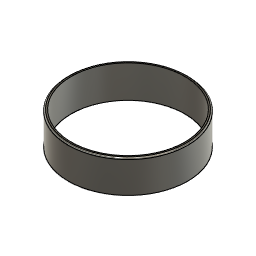
side v9 (Autodesk Fusion 360 design; units mm, degrees)
Autodesk Fusion 360 part; units mm, degrees
sketch "Sketch3" plane through (0, 0, 0) normal (0, 1, 0) x (1, 0, 0)
  circle A0 centre (0, 0) radius 40.3
  circle A1 centre (0, 0) radius 42.3
  line L0 (30, -20) -> (-30, -20)
  line L1 (-30, -20) -> (-30, 20)
  line L2 (-30, 20) -> (30, 20)
  line L3 (30, 20) -> (30, -20)
  line L4 (30, -20) -> (-30, 20) construction
  line L5 (-30, -20) -> (30, 20) construction
  dimension "d13" = 80.6
  dimension "d14" = 2
  dimension "d34" = 60
  dimension "d35" = 40
  constraint coincident A0.centre A1.centre
  constraint perpendicular L0 L1
  constraint parallel L0 L2
  constraint parallel L1 L3
  constraint horizontal L0
  constraint coincident L4 A0.centre
  constraint coincident L5 A0.centre
  measures "d13" diameter of A0
  measures "d34" distance of L1.end L2.end
  measures "d35" distance of L0.end L1.end
extrude "Extrude3" add sketch "Sketch3" along normal blind 21 contours A1
sketch "Sketch4" plane through (0, 0, 0) normal (0, 0, 1) x (1, 0, 0)
  line L0 (-49.5, 21) -> (-47.3, 21)
  line L1 (49.5, 21) -> (47.3, 21)
  line L2 (-47.3, 21) -> (-47.3, 25.1334)
  line L3 (47.3, 21) -> (47.3, 25.1334)
  line L4 (47.3, 27) -> (47.3, 25)
  arc A0 (47.3, 25) -> (-47.3, 25) centre (0, -131.3064) ccw
  line L5 (47.3, 21) -> (45.3, 21)
  line L6 (45.3, 21) -> (45.3, 25.5913)
  line L7 (-47.3, 21) -> (-45.3, 21)
  line L8 (-45.3, 21) -> (-45.3, 25.5913)
  arc A1 (0, 32) -> (-47.3, 25) centre (0, -131.3064) ccw
  line L9 (0, 32) -> (0, 34)
  arc A2 (45.4965, 27.5344) -> (-45.4965, 27.5344) centre (0, -129.3064) ccw
  arc A3 (-45.4965, 27.5344) -> (-47.3, 25.1334) centre (-44.8, 25.1334) ccw
  arc A4 (47.3, 25.1334) -> (45.4965, 27.5344) centre (44.8, 25.1334) ccw
  line L10 (0, 21) -> (-2.5, 21)
  line L11 (-2.5, 21) -> (-2.5, 31.9809)
  line L12 (0, 21) -> (0, 32)
  line L13 (-42, 21) -> (-39.8, 21)
  line L14 (42, 21) -> (39.8, 21)
  line L15 (39.8, 21) -> (39.8, 27.0759)
  line L16 (-39.8, 21) -> (-39.8, 27.0759)
  line L17 (-39.8, 21) -> (-37.8, 21)
  line L18 (-37.8, 21) -> (-37.8, 27.5651)
  line L19 (37.8, 21) -> (37.8, 27.5651)
  line L20 (37.8, 21) -> (39.8, 21)
  line L21 (-39.8, 27.0759) -> (-39.8, 29.0759)
  line L22 (39.8, 27.0759) -> (39.8, 29.0759)
  line L23 (-39.8, 27.0759) -> (0, 27.0759)
  line L24 (0, 27.0759) -> (0, 34)
  point P0 (-47.3, 27)
  dimension "d17" = 2.2
  dimension "d18" = 2.2
  dimension "d19" = 6
  dimension "d20" = 6
  dimension "d22" = 2
  dimension "d23" = 2
  dimension "d24" = 2
  dimension "d25" = 2
  dimension "d26" = 2
  dimension "d27" = 2.5
  dimension "d28" = 2.5
  dimension "d36" = 2.2
  dimension "d37" = 2.2
  dimension "d38" = 2
  dimension "d39" = 2
  constraint horizontal L0
  constraint horizontal L1
  constraint perpendicular L0 L2
  constraint perpendicular L1 L3
  constraint coincident L2 A0.end
  constraint coincident A1.start A0
  constraint perpendicular L3 L5
  constraint coincident A0 L6.end
  constraint perpendicular L5 L6
  constraint perpendicular L2 L7
  constraint coincident A0 L8.end
  constraint perpendicular L7 L8
  constraint vertical L9
  constraint coincident L9.end A2
  constraint coincident P0 L2
  constraint coincident P0 A2
  constraint tangent L2 A3
  constraint tangent A2 A3
  constraint coincident L4.start L3
  constraint coincident L4.start A2
  constraint tangent L3 A4
  constraint tangent A2 A4
  constraint equal A3 A4
  constraint horizontal L10
  constraint vertical L11
  constraint coincident A0 L11.end
  constraint coincident A1 L11.end
  constraint perpendicular L10 L12
  constraint horizontal L13
  constraint horizontal L14
  constraint coincident A0 L15.end
  constraint perpendicular L14 L15
  constraint vertical L16
  constraint coincident A0 L16.end
  constraint perpendicular L16 L17
  constraint vertical L18
  constraint coincident A0 L18.end
  constraint vertical L19
  constraint coincident A0 L19.end
  constraint perpendicular L15 L20
  constraint coincident A2 L21.end
  constraint vertical L21
  constraint coincident A2 L22.end
  constraint parallel L15 L22
  constraint coincident L12 L23.end
  constraint perpendicular L12 L23
  measures "d17" distance of L0.start L0.end
  measures "d18" distance of L1.start L1.end
  measures "d19" distance of L0.end P0
  measures "d20" distance of L1.end L4.start
  measures "d22" distance of L4.start L4.end
  measures "d23" distance of P0 A0.end
  measures "d24" distance of L1.end L5.end
  measures "d25" distance of L0.end L7.end
  measures "d26" distance of A1.start L9.end
  measures "d27" radius of A3
  measures "d28" distance of L10.start L10.end
  measures "d36" distance of L13.start L13.end
  measures "d37" distance of L14.start L14.end
  measures "d38" distance of L13.end L17.end
  measures "d39" distance of L14.end L19.start
sketch "Sketch5" plane through (0, 0, 0) normal (0, -1, 0) x (1, 0, 0)
  circle A0 centre (0, 0) radius 40.3
  circle A1 centre (0, 0) radius 42.3
extrude "Extrude4" add sketch "Sketch5" along normal blind 2 contours A0 | A1
fillet "Fillet2" radius 1 1 edges at (-39.4374, 21, 15.2963)
sketch "Sketch6" plane through (0, -2, 0) normal (0, -1, 0) x (1, 0, 0)
  line L0 (20, 27.5) -> (-20, 27.5)
  line L1 (-20, 27.5) -> (-20, -27.5)
  line L2 (-20, -27.5) -> (20, -27.5)
  line L3 (20, -27.5) -> (20, 27.5)
  line L4 (20, 27.5) -> (-20, -27.5) construction
  line L5 (-20, 27.5) -> (20, -27.5) construction
  circle A0 centre (0, 0) radius 42.3
  dimension "d41" = 55
  dimension "d42" = 40
  constraint perpendicular L0 L1
  constraint parallel L0 L2
  constraint parallel L1 L3
  constraint horizontal L0
  constraint coincident L4 A0.centre
  constraint coincident L5 A0.centre
  measures "d41" distance of L0.end L1.end
  measures "d42" distance of L1.end L2.end
sketch "Sketch7" plane through (0, -2, 0) normal (0, -1, 0) x (1, 0, 0)
  circle A0 centre (0, 0) radius 42.3
sketch "Sketch8" plane through (0, -2, 0) normal (0, -1, 0) x (1, 0, 0)
  circle A0 centre (0, 0) radius 42.3
sketch "Sketch9" plane through (0, 0, 0) normal (0, 0, 1) x (1, 0, 0)
sketch "Sketch10" plane through (0, -2, 0) normal (0, -1, 0) x (1, 0, 0)
  circle A0 centre (0, 0) radius 42.3
  circle A1 centre (0, 0) radius 40.3
  dimension "d43" = -2
extrude "Extrude5" cut sketch "Sketch10" against normal blind 3 contours A1
sketch "Sketch11" plane through (0, 21, 0) normal (0, 1, 0) x (-1, 0, 0)
  circle A0 centre (0, 0) radius 40.3
  circle A1 centre (0, 0) radius 41.3
  line L0 (42, 0) -> (40.3, 0)
  line L1 (40.3, 0) -> (39.3, 0)
  circle A2 centre (0, 0) radius 39.3
  dimension "d46" = 1
  constraint coincident A0 L0.end
  constraint horizontal L0
  constraint horizontal L1
  constraint concentric A0 A2
  constraint coincident L1.end A2
  measures "d46" distance of L0.end L1.end
extrude "Extrude6" [suppressed]
fillet "Fillet3" [suppressed]
equation "d17 = 2 mm + 0.2 mm"
equation "d18 = 2 mm + 0.2 mm"
equation "d36 = 2 mm + 0.2 mm"
equation "d37 = 2 mm + 0.2 mm"
